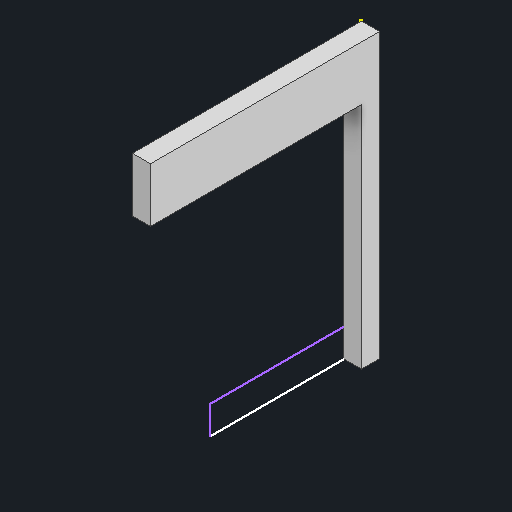
# Autodesk Inventor part: e
Saved by Autodesk Inventor 2024 (Build 280153000, 153)
## iProperties
Created: 2023-06-10
Part Number: e
Material: Generic
Document SubType Name: Modeling
Designer: pc
Density: 1 g/cm^3
Appearance: Default
Author: pc
Autodesk Inventor part; units mm, degrees
ref_plane "YZ Plane" through (0, 0, 0) normal (1, 0, 0) x (0, 1, 0)
ref_plane "XZ Plane" through (0, 0, 0) normal (0, 1, 0) x (-1, 0, 0)
ref_plane "XY Plane" through (0, 0, 0) normal (0, 0, 1) x (1, 0, 0)
sketch "Sketch1" plane through (0, 0, 0) normal (0, 0, 1) x (1, 0, 0)
  line L0 (0, 0) -> (7.62, 0)
  line L1 (7.62, 0) -> (7.62, -22.86)
  line L2 (7.62, -22.86) -> (0, -22.86)
  line L3 (0, -22.86) -> (0, 0)
  line L4 (7.62, -22.86) -> (0, -22.86)
  line L5 (0, -22.86) -> (0, -119.38)
  line L6 (0, -119.38) -> (7.62, -119.38)
  line L7 (7.62, -119.38) -> (7.62, -22.86)
  line L8 (0, -111.76) -> (0, -119.38)
  line L9 (0, 0) -> (7.62, 0)
  line L10 (7.62, 0) -> (7.62, -22.86)
  line L11 (7.62, -22.86) -> (0, -22.86)
  line L12 (0, -22.86) -> (0, 0)
  line L13 (7.62, -119.38) -> (35.0744, -119.38)
  line L14 (35.0744, -119.38) -> (69.9139, -119.38)
  line L15 (69.9139, -111.76) -> (69.9139, -119.38)
  line L16 (69.9139, -111.76) -> (7.62, -111.76)
  point P0 (0, -22.86)
  dimension "d0" = 7.62
  dimension "d1" = 22.86
  dimension "d2" = 7.62
  dimension "d3" = 96.52
  dimension "d6" = 7.62
  constraints: 34 end point, 7 parallel, 3 horizontal, 3 perpendicular, 3 point on line
  measures "d0" distance of L1.end L2.end
  measures "d1" distance of L0.end L1.end
  measures "d2" distance of L6.end L5.end
  measures "d3" distance of L5.end L4.end
  measures "d6" distance of L10.end L11.end
extrude "Extrusion1" add sketch "Sketch1" along normal blind 7.62 contours L0 L1 L2 L3 | L2 L7 L6 L5
extrude "Extrusion2" add sketch "Sketch1" along normal blind 96.52 contours L0 L1 L2 L3
sketch "Sketch2" plane through (0, -119.38, 0) normal (-1, 0, 0) x (0, 0, 1)
  line L0 (0, 0) -> (7.62, 0) projected
  line L1 (7.62, 0) -> (63.8725, 0)
  line L2 (63.8725, 0) -> (63.8725, 11.8579)
  line L3 (63.8725, 11.8579) -> (7.62, 11.8579)
  point P0 (0, 119.38)
  constraints: 6 end point, 2 perpendicular, 1 horizontal
equation "\"d0\" = d6"
body "Solid1"
